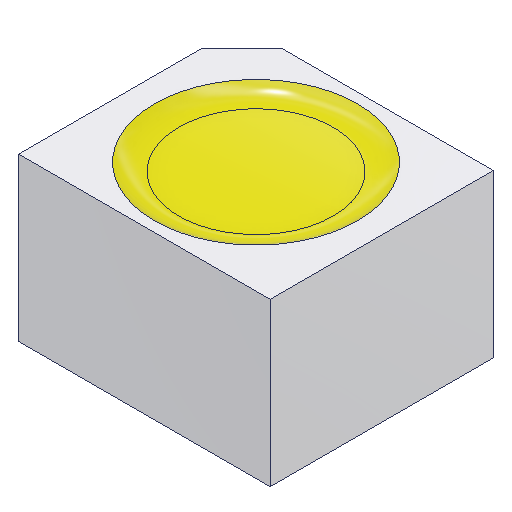
# Autodesk Inventor part: led od paska ledów
Saved by Autodesk Inventor 2026.1 (Build 301233000, 233)
## iProperties
Created: 2016-06-18
Part Number: led od paska ledów
Material: Ogólny
Document SubType Name: Modeling
Designer: Andrzej
Density: 1 g/cm^3
Appearance: PTFE
Mass: 0.0163798 g
Surface Area: 0.397755 cm^2
Volume: 0.0163798 cm^3
Author: Andrzej
Autodesk Inventor part; units mm, degrees
ref_plane "YZ Plane" through (0, 0, 0) normal (1, 0, 0) x (0, 1, 0)
ref_plane "XZ Plane" through (0, 0, 0) normal (0, 1, 0) x (-1, 0, 0)
ref_plane "XY Plane" through (0, 0, 0) normal (0, 0, 1) x (1, 0, 0)
sketch "Szkic1" plane through (0, 0, 0) normal (0, 0, 1) x (1, 0, 0)
  line L0 (-1.55, 1.375) -> (1.55, 1.375)
  line L1 (1.55, 1.375) -> (1.55, -1.375)
  line L2 (1.55, -1.375) -> (-1.55, -1.375)
  line L3 (-1.55, -1.375) -> (-1.55, 1.375)
  point P0 (0, 0)
  dimension "d0" = 3.1
  dimension "d1" = 2.75
  dimension "d15" = 1.375
  dimension "d16" = 1.55
  constraints: 8 end point, 2 parallel, 1 horizontal, 1 perpendicular
  measures "d0" distance of L1.end L2.end
  measures "d1" distance of L0.end L1.end
  measures "d15" distance from line of L0 point (0, 0)
  measures "d16" distance from line of L3 point (0, 0)
extrude "Wyciągnięcie proste1" add sketch "Szkic1" along normal blind 2
chamfer "Faza1" distance 0.5 angle 45 1 edges at (-1.55, 1.375, 1)
sketch "Szkic2" plane through (0, 0, 2) normal (0, 0, 1) x (1, 0, 0)
  line L0 (1.55, 1.375) -> (-1.05, 1.375) projected
  line L1 (-1.55, -1.375) -> (1.55, -1.375) projected
  line L2 (-1.55, 0.875) -> (-1.55, -1.375) projected
  circle A0 centre (0, 0) radius 1.25
  point P0 (0, 0)
  dimension "d7" = 2.75
  dimension "d8" = 1.375
  dimension "d9" = 3.1
  dimension "d10" = 1.55
  dimension "d11" = 2.5
  constraints: 1 centre point, 1 coincident
  measures "d7" distance between parallel lines of L0 L1
  measures "d8" distance from line of L1 point (0, 0)
  measures "d9" distance of L1.start L1.end
  measures "d10" distance from line of L2 point (0, 0)
  measures "d11" diameter of A0
extrude "Wyciągnięcie proste2" cut sketch "Szkic2" against normal blind 0.1
fillet "Zaokrąglenie1" radius 0.5 1 edges at (-1.25, 0, 1.9)
equation "\"d15\" = 0.5 * d1"
equation "\"d16\" = 0.5 * d0"
equation "\"d8\" = 0.5 * d7"
equation "\"d10\" = 0.5 * d9"
